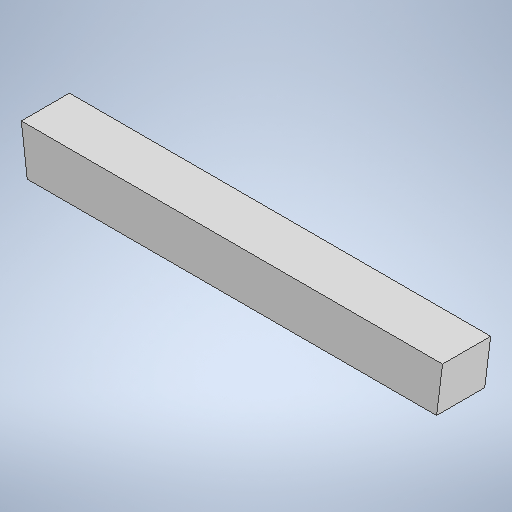
# Autodesk Inventor part: Lid_Divider
Saved by Autodesk Inventor 2025 (Build 290162010, 162A)
## iProperties
Created: 2024-10-17
Part Number: Lid_Divider
Material: Generic
Document SubType Name: Modeling
Designer: vncnt
Density: 1 g/cm^3
Appearance: Default
Author: vncnt
Autodesk Inventor part; units mm, degrees
ref_plane "YZ Plane" through (0, 0, 0) normal (1, 0, 0) x (0, 1, 0)
ref_plane "XZ Plane" through (0, 0, 0) normal (0, 1, 0) x (-1, 0, 0)
ref_plane "XY Plane" through (0, 0, 0) normal (0, 0, 1) x (1, 0, 0)
sketch "Sketch1" plane through (0, 0, 0) normal (0, 0, 1) x (1, 0, 0)
  line L0 (-107.95, 25.4) -> (107.95, 25.4)
  line L1 (107.95, 25.4) -> (107.95, -25.4)
  line L2 (107.95, -25.4) -> (-107.95, -25.4)
  line L3 (-107.95, -25.4) -> (-107.95, 25.4)
  line L4 (-107.95, 25.4) -> (107.95, -25.4) construction
  line L5 (107.95, 25.4) -> (-107.95, -25.4) construction
  line L6 (0, 25.4) -> (114.3, 25.4)
  line L7 (114.3, 25.4) -> (107.95, -25.4)
  line L8 (0, 25.4) -> (-114.3, 25.4)
  line L9 (-114.3, 25.4) -> (-107.95, -25.4)
  line L10 (-107.95, 25.4) -> (107.95, 25.4)
  line L11 (107.95, 25.4) -> (107.95, 27.5463)
  line L12 (107.95, 27.5463) -> (-107.95, 27.5463)
  line L13 (-107.95, 27.5463) -> (-107.95, 25.4)
  point P0 (0, 0)
  point P1 (107.95, 25.4)
  point P2 (-107.95, 25.4)
  dimension "d0" = 215.9
  dimension "d1" = 50.8
  dimension "d2" = 114.3
  dimension "d3" = 114.3
  dimension "d4" = 2.1463
  constraints: 28 end point, 3 horizontal, 3 midpoint, 3 parallel, 2 perpendicular, 1 point on line
  measures "d0" distance of L1.end L2.end
  measures "d1" distance of L0.end L1.end
  measures "d2" distance of L6.start L6.end
  measures "d3" distance of L6.start L8.end
  measures "d4" distance of L11.end L10.end
extrude "Extrusion1" add sketch "Sketch1" along normal blind 25.4
sketch "Sketch2" plane through (0, 0, 25.4) normal (0, 0, 1) x (1, 0, 0)
  line L0 (-120.0424, 48.8596) -> (122.5706, 48.8596)
  line L1 (122.5706, 48.8596) -> (122.5706, -0.3726)
  line L2 (122.5706, -0.3726) -> (-120.0424, -0.3726)
  line L3 (-120.0424, -0.3726) -> (-120.0424, 48.8596)
  point P0 (0, 0)
  constraints: 8 end point, 2 parallel, 1 horizontal, 1 perpendicular
extrude "Extrusion2" cut sketch "Sketch2" against normal through all
body "Solid1"
